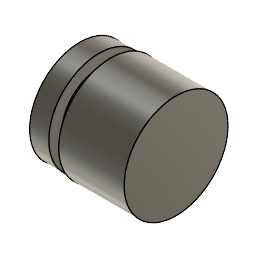
Turning (Autodesk Fusion 360 design; units mm, degrees)
part number: 2026-06-24-20-04-57-179
Autodesk Fusion 360 part; units mm, degrees
sketch "Sketch1" plane through (0, 0, 0) normal (0, 1, 0) x (1, 0, 0)
  line L0 (0, 0) -> (100, 0)
  line L1 (0, 0) -> (0, -52.2578)
  line L2 (0, -52.2578) -> (20, -52.2578)
  line L3 (20, -52.2578) -> (20, -39)
  line L4 (20, -39) -> (32, -39)
  line L5 (32, -39) -> (32, -54)
  line L6 (32, -54) -> (100, -54)
  line L7 (100, -54) -> (100, 0)
  dimension "d1" = 20
  dimension "d2" = 12
  dimension "d4" = 78
  dimension "d5" = 108
  constraint coincident L0.start L1.start
  constraint horizontal L0
  constraint perpendicular L0 L1
  constraint perpendicular L1 L2
  constraint perpendicular L2 L3
  constraint perpendicular L1 L4
  constraint parallel L4 L6
  constraint perpendicular L0 L7
  measures "d1" distance of L1.end L2.end
  measures "d2" distance of L3.end L4.end
revolve "Revolve1" add sketch "Sketch1" angle 360 about axis through (0, 0, 0) along (1, 0, 0)
